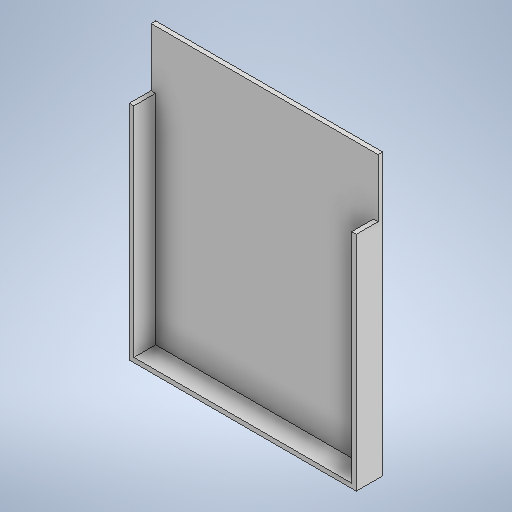
# Autodesk Inventor part: back
Saved by Autodesk Inventor 2025 (Build 290162000, 162)
## iProperties
Created: 2024-11-13
Part Number: back
Material: Generic
Document SubType Name: Modeling
Designer: ethan
Density: 1 g/cm^3
Appearance: Default
Author: ethan
Autodesk Inventor part; units mm, degrees
ref_plane "YZ Plane" through (0, 0, 0) normal (1, 0, 0) x (0, 1, 0)
ref_plane "XZ Plane" through (0, 0, 0) normal (0, 1, 0) x (-1, 0, 0)
ref_plane "XY Plane" through (0, 0, 0) normal (0, 0, 1) x (1, 0, 0)
sketch "Sketch1" plane through (0, 0, 0) normal (0, 1, 0) x (-1, 0, 0)
  line L0 (0, 0) -> (95.25, 0)
  line L1 (95.25, 0) -> (95.25, -9.525)
  line L2 (95.25, -9.525) -> (0, -9.525)
  line L3 (0, -9.525) -> (0, 0)
  line L4 (-2, -11.525) -> (97.25, -11.525)
  line L5 (97.25, -11.525) -> (97.25, 2)
  line L6 (97.25, 2) -> (-2, 2)
  line L7 (-2, 2) -> (-2, -11.525)
  line L8 (95.25, 0) -> (97.25, 0)
  line L9 (0, 0) -> (-2, 0)
  dimension "d0" = 95.25
  dimension "d1" = 9.525
  dimension "d4" = 2
  constraints: 20 end point, 4 parallel, 3 perpendicular, 3 point on line, 1 horizontal, 3 other
  measures "d0" distance of L1.end L2.end
  measures "d1" distance of L0.end L1.end
  measures "d4" distance between parallel lines of L2 L4
extrude "Extrusion1" add sketch "Sketch1" along normal blind 2 contours L0 L1 L2 L3 | L3 L2 L1 L8 L5 L4 L7 L9
sketch "Sketch2" plane through (0, 2, 0) normal (0, 1, 0) x (1, 0, 0)
  line L0 (-97.25, 0) -> (2, 0) projected
  line L1 (2, 0) -> (2, 11.525) projected
  line L2 (2, 11.525) -> (-97.25, 11.525) projected
  line L3 (-97.25, 11.525) -> (-97.25, 0) projected
  line L4 (0, 9.525) -> (0, 2)
  line L5 (0, 2) -> (-95.25, 2)
  line L6 (-95.25, 2) -> (-95.25, 9.525)
  line L7 (-95.25, 9.525) -> (0, 9.525)
  line L8 (0, 2) -> (0, 0)
  line L9 (-95.25, 2) -> (-95.25, 0)
  dimension "d5" = 2
  constraints: 12 end point, 1 perpendicular, 1 point on line, 3 other
  measures "d5" distance between parallel lines of L1 L4
extrude "Extrusion2" add sketch "Sketch2" along normal blind 95.25 contours L3 L2 L1 L0 L8 L4 L7 L6 L9
sketch "Sketch3" plane through (0, 97.25, 0) normal (0, 1, 0) x (1, 0, 0)
  line L0 (-97.25, 0) -> (-95.25, 0) projected
  line L1 (-95.25, 0) -> (-95.25, 9.525) projected
  line L2 (-95.25, 9.525) -> (0, 9.525) projected
  line L3 (0, 9.525) -> (0, 0) projected
  line L4 (0, 0) -> (2, 0) projected
  line L5 (2, 0) -> (2, 11.525) projected
  line L6 (2, 11.525) -> (-97.25, 11.525) projected
  line L7 (-97.25, 11.525) -> (-97.25, 0) projected
  line L8 (-97.25, 11.525) -> (2, 11.525)
  line L9 (2, 11.525) -> (2, 9.525)
  line L10 (2, 9.525) -> (-97.25, 9.525)
  line L11 (-97.25, 9.525) -> (-97.25, 11.525)
  dimension "d8" = 99.25
  constraints: 8 end point, 2 parallel, 1 horizontal, 1 perpendicular, 1 point on line
  measures "d8" distance of L9.end L10.end
extrude "Extrusion3" add sketch "Sketch3" along normal blind 25.4 contours L7 L6 L5 L10 L2
body "Solid1"
